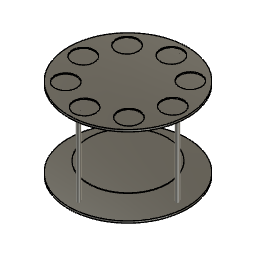
Alkohol Karusel v1 (Autodesk Fusion 360 design; units mm, degrees)
Autodesk Fusion 360 part; units mm, degrees
sketch "Sketch1" plane through (0, 0, 0) normal (0, 0, 1) x (1, 0, 0)
  circle A0 centre (0, 0) radius 30
  dimension "d1" = 60
  constraint coincident A0.centre origin
  measures "d1" diameter of A0
extrude "Extrude1" add sketch "Sketch1" along normal blind 1 makes body 1
copy_body "CopyPasteBodies1" bodies 1 makes body 2
move_body "Move1" bodies 2 to x (1, 0, 0) y (0, 1, 0) z (0, 0, 1) at (0, 0, 0)
move_body "Move2" bodies 2 to x (1, 0, 0) y (0, 1, 0) z (0, 0, 1) at (0, 0, 40)
sketch "Sketch2" plane through (0, 0, 41) normal (0, 0, 1) x (-1, 0, 0)
  circle A0 centre (0, 0) radius 30
  circle A1 centre (-25, -50) radius 20
  dimension "d4" = 40
  measures "d4" diameter of A1
extrude "Extrude2" add sketch "Sketch2" along normal blind 0.2 separate body contours A1 makes body 3
move_body "Move3" bodies 3 to x (1, 0, 0) y (0, 1, 0) z (0, 0, 1) at (-25, -50, -35)
sketch "Sketch3" plane through (0, 0, 0) normal (0, 0, 1) x (1, 0, 0)
  circle A0 centre (0, 40) radius 1
  dimension "d7" = 2
  measures "d7" diameter of A0
extrude "Extrude3" add sketch "Sketch3" along normal blind 40 separate body makes body 4
copy_body "CopyPasteBodies2" bodies 4 makes body 5
move_body "Move4" bodies 5 to x (1, 0, 0) y (0, 1, 0) z (0, 0, 1) at (0, 0, 0)
move_face "MoveFace1" to x (1, 0, 0) y (0, 1, 0) z (0, 0, 1) at (0, -15, 0) 1 faces at (-0.9397, 39.658, 26.6667) on bodies 4
move_body "Move5" bodies 5 to x (1, 0, 0) y (0, 1, 0) z (0, 0, 1) at (0, -65, 0)
copy_body "CopyPasteBodies3" bodies 4 makes body 6
copy_body "CopyPasteBodies4" bodies 4 makes body 7
move_body "Move6" bodies 7 to x (1, 0, 0) y (0, 1, 0) z (0, 0, 1) at (25, -25, 0)
copy_body "CopyPasteBodies5" bodies 4 makes body 8
move_body "Move7" bodies 8 to x (1, 0, 0) y (0, 1, 0) z (0, 0, 1) at (-25, -25, 0)
sketch "Sketch4" plane through (0, 0, 41) normal (0, 0, 1) x (-1, 0, 0)
  circle A0 centre (0, 0) radius 30
  circle A1 centre (-0.3343, 22.2962) radius 5.5
  dimension "d10" = 11
  measures "d10" diameter of A1
extrude "Extrude4" cut sketch "Sketch4" against normal blind 0.5 contours A1 bodies 2
pattern_circular "C-Pattern1" count 8 over 360 about axis through (0, 0, 1.75) along (0, 0, 1) of "Extrude4"
